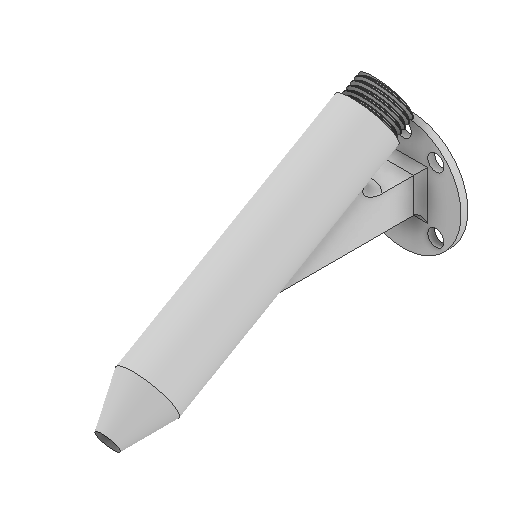
# Autodesk Inventor part: MountingFlange
Saved by Autodesk Inventor 2025.2 (Build 292293000, 293)
## iProperties
Created: 2025-09-05
Part Number: MountingFlange
Material: Genérico
Document SubType Name: Modeling
Designer: Lab Geotecnia
Density: 1 g/cm^3
Appearance: Valor por defecto
Checked By: Mateo Ramos
Author: Jeison Nicolas Diaz Arciniegas
Title: Herramienta de dibujo
Autodesk Inventor part; units mm, degrees
ref_plane "YZ Plane" through (0, 0, 0) normal (1, 0, 0) x (0, 1, 0)
sketch "Boceto1" plane through (0, 0, 0) normal (0, 0, 1) x (1, 0, 0)
  line L0 (-4547.1855, 0) -> (6211.9028, 0) construction
  line L1 (0, 1530.4936) -> (0, -2289.0976) construction
  circle A0 centre (0, 0) radius 25
  circle A1 centre (0, 0) radius 20 construction
  circle A2 centre (0, 0) radius 12.5
  line L2 (0, 0) -> (-32.1909, 32.1909) construction
  line L3 (0, 0) -> (26.6923, 26.6923) construction
  circle A3 centre (0, 20) radius 3.5
  circle A4 centre (-14.1421, 14.1421) radius 3.5
  circle A5 centre (14.1421, 14.1421) radius 3.5
  line L4 (0, 0) -> (-27.9428, -27.9428) construction
  circle A6 centre (-14.1421, -14.1421) radius 3.5
  line L5 (0, 0) -> (27.9428, -27.9428) construction
  circle A7 centre (14.1421, -14.1421) radius 3.5
  dimension "d1" = 50
  dimension "d3" = 40
  dimension "d4" = 25
  dimension "d5" = 45
  dimension "d6" = 45
  dimension "d8" = 7
  dimension "d9" = 7
  dimension "d10" = 7
  dimension "d11" = 45
  dimension "d12" = 7
  constraints: 12 end point, 8 centre point, 5 point on line, 4 point on circle, 3 coincident, 2 horizontal, 2 symmetric about line, 2 vertical, 2 other
  measures "d1" diameter of A0
  measures "d3" diameter of A1
  measures "d4" diameter of A2
  measures "d5" angle of L1 L2
  measures "d6" angle of L1 L3
  measures "d8" diameter of A3
  measures "d9" diameter of A4
  measures "d10" diameter of A5
  measures "d11" angle of L0 L4
  measures "d12" diameter of A6
extrude "Extrusion1" add sketch "Boceto1" along normal blind 3
sketch "Sketch5" plane through (0, 0, 3) normal (0, 0, 1) x (1, 0, 0)
  circle A0 centre (0, 0) radius 12.5 projected
  circle A1 centre (0, 0) radius 12.5
  constraints: 1 centre point, 1 coincident
extrude "Extrusion7" add sketch "Sketch5" against normal blind 3
sketch "Sketch17" plane through (0, 0, 0) normal (0, 1, 0) x (-1, 0, 0)
  line L0 (25, 3) -> (-25, 3) projected
  line L1 (0, 3) -> (0, 73)
  point P0 (0, 0)
  dimension "d70" = 70
  constraints: 2 end point, 1 midpoint, 1 vertical
  measures "d70" distance of L1.start L1.end
ref_plane "Work Plane2" through (0, 0, 70) normal (0, 0, 1) x (1, 0, 0)
sketch "Sketch18" plane through (0, 0, 70) normal (0, 0, 1) x (1, 0, 0)
  line L0 (-35.3975, 0) -> (46.7248, 0)
  point P0 (0, 0)
  constraints: 2 end point, 1 horizontal
ref_plane "Work Plane3" through (-35.3975, 0, 70) normal (0, -0.5, 0.8660254) x (1, 0, 0)
sketch "Sketch19" plane through (-35.3975, 0, 70) normal (0, -0.5, 0.8660254) x (1, 0, 0)
  circle A0 centre (35.3975, 1.5) radius 9
  circle A1 centre (35.3975, 1.5) radius 12.5
  point P0 (35.3975, -35)
  dimension "d73" = 18
  dimension "d74" = 25
  constraints: 2 centre point, 2 coincident
  measures "d73" diameter of A0
  measures "d74" diameter of A1
extrude "Extrusion13" add sketch "Sketch19" along normal blind 50 and the other way blind 60
sketch "Sketch20" plane through (0, 0, 3) normal (0, 0, 1) x (1, 0, 0)
  line L0 (-7.5, -7.5) -> (7.5, -7.5)
  line L1 (7.5, -7.5) -> (7.5, 7.5)
  line L2 (7.5, 7.5) -> (-7.5, 7.5)
  line L3 (-7.5, 7.5) -> (-7.5, -7.5)
  circle A0 centre (0, 0) radius 12.5 projected
  line L4 (-7.5, -7.5) -> (7.5, 7.5) construction
  line L5 (7.5, -7.5) -> (-7.5, 7.5) construction
  dimension "d79" = 15
  dimension "d80" = 15
  constraints: 12 end point, 2 midpoint, 2 parallel, 1 horizontal, 1 perpendicular
  measures "d79" distance of L2.end L1.end
  measures "d80" distance of L1.end L0.end
extrude "Extrusion14" add sketch "Sketch20" along normal up to next contours L3 L2 L1 L0
ref_plane "Work Plane4" through (-35.3975, -30, 121.9615) normal (0, -0.5, 0.8660254) x (1, 0, 0)
sketch "Sketch22" plane through (-35.3975, -30, 121.9615) normal (0, -0.5, 0.8660254) x (1, 0, 0)
  circle A0 centre (35.3975, 1.5) radius 2.5
  point P0 (35.3975, -35)
  dimension "d90" = 5
  constraints: 1 centre point, 1 coincident
  measures "d90" diameter of A0
sketch "Sketch23" plane through (0, -23.701, 114.0513) normal (0, -0.5, 0.8660254) x (1, 0, 0)
  circle A0 centre (0, 0) radius 12.5 projected
  point P0 (0, -36.5)
ref_plane "Work Plane5" through (-35.3975, -35, 130.6218) normal (0, -0.5, 0.8660254) x (1, 0, 0)
sketch "Sketch33" plane through (-35.3975, -35, 130.6218) normal (0, -0.5, 0.8660254) x (1, 0, 0)
  circle A0 centre (35.3975, 1.5) radius 5
  point P0 (35.3975, -35)
  dimension "d143" = 10
  constraints: 1 centre point, 1 coincident
  measures "d143" diameter of A0
loft "Loft3" add profiles "Sketch33" section 1 edges at (-12.5, -23.701, 114.0513)
sketch "Sketch34" plane through (0, 0, 0) normal (1, 0, 0) x (0, 1, 0)
  line L0 (-12.8756, 120.3013) -> (-29.3708, 133.8718) projected
  line L1 (-12.8756, 120.3013) -> (-34.5263, 107.8013) projected
  line L2 (-38.0311, 128.8718) -> (-29.3708, 133.8718) projected
  line L3 (-15.9067, 118.5513) -> (39.0933, 23.2885) projected
  line L4 (-31.4952, 109.5513) -> (23.5048, 14.2885) projected
  line L5 (-29.3708, 133.8718) -> (-33.701, 131.3718)
  line L6 (-38.0311, 128.8718) -> (-29.3708, 133.8718) projected
  line L7 (-33.701, 131.3718) -> (52.8084, -18.4669)
  line L8 (-15.9067, 118.5513) -> (-29.3708, 133.8718)
  line L9 (-29.3708, 133.8718) -> (-33.701, 131.3718)
  point P0 (0, 0)
  point P1 (-23.701, 114.0513)
  dimension "d148" = 5
  constraints: 8 end point, 2 parallel, 1 collinear, 1 midpoint
  measures "d148" distance of L2.end L5.end
revolve "Revolution6" cut sketch "Sketch34" angle 360 about axis through (0, -33.701, 131.3718) along (0, 0.5, -0.8660254) contours L8 L1 L7 L2
sketch "Sketch35" plane through (0, 31.299, 18.7885) normal (0, 0.5, -0.8660254) x (-1, 0, 0)
  circle A0 centre (0, 0) radius 9 projected
  circle A1 centre (0, 0) radius 12.5 projected
  circle A2 centre (0, 0) radius 9
  circle A3 centre (0, 0) radius 10
  point P0 (0, -36.5)
  dimension "d150" = 20
  constraints: 2 centre point, 2 coincident, 1 concentric
  measures "d150" diameter of A3
extrude "Extrusion17" add sketch "Sketch35" along normal blind 10 contours A3
sketch "Sketch40" plane through (0, 36.299, 10.1282) normal (0, -0.8660254, -0.5) x (1, 0, 0)
  line L0 (10, 0) -> (10, 10)
  line L1 (10, 10) -> (8.1463, 10)
  line L2 (8.1463, 10) -> (8.1463, 0)
  line L3 (8.1463, 0) -> (10, 0)
  line L4 (0, -39.9031) -> (0, 178.0193) projected
  constraints: 8 end point
revolve "Revolution9" cut sketch "Sketch40" angle 360 about axis through (0, 36.299, 10.1282) along (0, -0.5, 0.8660254)
fillet "Fillet3" radius 3 4 edges at (0, 7.5, 3) (7.5, 0, 3) (0, -7.5, 3) (-7.5, 0, 3)
sketch "Sketch42" plane through (0, 31.299, 18.7885) normal (0, 0.5, -0.8660254) x (-1, 0, 0)
  circle A0 centre (0, 0) radius 9 projected
  circle A1 centre (0, 0) radius 9
  circle A2 centre (0, 0) radius 11
  point P0 (0, -36.5)
  dimension "d198" = 22
  constraints: 2 centre point, 2 coincident, 1 concentric
  measures "d198" diameter of A2
extrude "Extrusion18" add sketch "Sketch42" along normal blind 10
thread "Thread8" size "M22x2" class "6g" standard "ANSI Metric M Profile" full length
sketch "Sketch44" plane through (0, 36.299, 10.1282) normal (0, -0.8660254, -0.5) x (1, 0, 0)
  line L0 (11, 0) -> (11, 10)
  line L1 (11, 10) -> (9.5171, 10)
  line L2 (9.5171, 10) -> (9.5171, 0)
  line L3 (9.5171, 0) -> (11, 0)
  line L4 (0, -47.3353) -> (0, 189.2709) projected
  constraints: 8 end point
revolve "Revolution11" cut sketch "Sketch44" angle 360 about axis through (0, 36.299, 10.1282) along (0, -0.5, 0.8660254)
sketch "Sketch45" plane through (0, 36.299, 10.1282) normal (0, -0.8660254, -0.5) x (1, 0, 0)
  line L0 (11, 0) -> (11, 10)
  line L1 (11, 10) -> (9.5171, 10)
  line L2 (9.5171, 10) -> (9.5171, 0)
  line L3 (9.5171, 0) -> (11, 0)
  line L4 (0, -46.5648) -> (0, 189.1425) projected
  constraints: 8 end point
revolve "Revolution12" add sketch "Sketch45" angle 360 about axis through (0, 36.299, 10.1282) along (0, -0.5, 0.8660254) separate body
sketch "Sketch43" plane through (0, 36.299, 10.1282) normal (0, 0.8660254, 0.5) x (0, -0.5, 0.8660254)
  line L0 (-1.1668, -9.6184) -> (-1.0001, -9.6184) construction
  line L1 (0.1666, -10.899) -> (-0.0001, -11.2192) construction
  line L2 (-2.0001, -11.2192) -> (-2.1668, -10.899) construction
  line L3 (-0.8334, -9.6184) -> (-1.0001, -9.2982) construction
  line L4 (-1.0001, -9.2982) -> (-1.1668, -9.6184) construction
  line L5 (-2.0001, -11.2192) -> (-1.8334, -10.899) construction
  line L6 (-0.8334, -9.6184) -> (-0.1668, -10.899)
  line L7 (-2.1668, -10.899) -> (-1.8334, -10.899) construction
  arc A0 (-2.1668, -10.899) -> (-2.0001, -11.0002) centre (-2.0001, -10.8123) ccw construction
  line L8 (0.1666, -10.899) -> (-0.1668, -10.899) construction
  line L9 (-2.0001, -11.2192) -> (-2.0001, -10.899) construction
  line L10 (-0.0001, -11.2192) -> (-0.0001, -10.899) construction
  line L11 (-1.0001, -9.2982) -> (-1.0001, -9.5172) construction
  line L12 (-2.0001, -11.0002) -> (-0.0001, -11.0002)
  arc A1 (-2.0001, -11.0002) -> (-1.8334, -10.899) centre (-2.0001, -10.8123) ccw
  line L13 (-0.1668, -10.899) -> (-0.0001, -11.2192) construction
  line L14 (-1.8334, -10.899) -> (-1.1668, -9.6184)
  line L15 (-0.0001, -0.0002) -> (-0.0001, 0.0177)
  line L16 (-0.0001, 0.0177) -> (-0.0001, -0.0002)
  line L17 (-0.0001, -0.0002) -> (0.0334, -0.0002)
  arc A2 (-0.1668, -10.899) -> (-0.0001, -11.0002) centre (-0.0001, -10.8123) ccw
  arc A3 (-0.0001, -11.0002) -> (0.1666, -10.899) centre (-0.0001, -10.8123) ccw construction
  arc A4 (-1.0001, -9.5172) -> (-1.1668, -9.6184) centre (-1.0001, -9.7051) ccw
  arc A5 (-0.8334, -9.6184) -> (-1.0001, -9.5172) centre (-1.0001, -9.7051) ccw
  line L18 (-1.0001, -9.5172) -> (-1.0001, -9.6184) construction
  line L19 (-1.0001, -9.6184) -> (-0.8334, -9.6184) construction
  dimension "d203" = 55
  dimension "d204" = 0.3202
  dimension "d205" = 0.3202
  dimension "Sketch43_ThreadOffset" = 0
  dimension "Sketch43_MajorRadius" = 11
  dimension "d208" = 2
  dimension "Sketch43_MinorRadius" = 9.5171
  constraints: 40 end point, 12 point on circle, 10 parallel, 8 tangent, 6 centre point, 6 collinear, 2 midpoint, 2 point on line, 1 horizontal, 1 perpendicular, 3 other
  measures "d203" angle of L6 L14
  measures "d204" distance of L3.end L0.end
  measures "d205" distance of L1.end L10.end
  measures "Sketch43_ThreadOffset" distance between parallel lines of L15 L10
  measures "Sketch43_MajorRadius" distance from line of L12 L15.start
  measures "d208" distance from line of L1.end L9
  measures "Sketch43_MinorRadius" distance edge to line of A5 L17
coil "Coil5" sketch "Sketch43" operation cut axis through (0, 36.299, 10.1282) along (0, -0.5, 0.8660254) pitch 2.002 turns 6.993007 hand right bodies 2
fillet "Fillet4" radius 5 1 edges at (0, 7.5, 35.0096)
equation "\"d203\" = d210"
equation "\"d204\" = 0.160083 * Sketch43_Pitch"
equation "\"d205\" = 0.160083 * Sketch43_Pitch"
equation "\"d208\" = Sketch43_Pitch"
equation "\"d108\" = 55deg"
equation "\"Sketch26_Pitch\" = 1.5"
equation "\"d129\" = 55deg"
equation "\"Sketch29_Pitch\" = 1"
equation "\"d162\" = 55deg"
equation "\"Sketch36_Pitch\" = 1"
equation "\"d185\" = 55deg"
equation "\"Sketch39_Pitch\" = 2.5"
equation "\"d210\" = 55deg"
equation "\"Sketch43_Pitch\" = 2"
body "Solid1"
body "Solid6"
